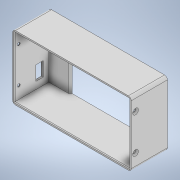
# Autodesk Inventor part: screen cover
Saved by Autodesk Inventor 2021 (Build 250183000, 183)
## iProperties
Created: 2022-01-29
Part Number: screen cover
Material: Generic
Document SubType Name: Modeling
Designer: Toby
Density: 1 g/cm^3
Appearance: Default
Author: Toby
Autodesk Inventor part; units mm, degrees
ref_plane "YZ Plane" through (0, 0, 0) normal (1, 0, 0) x (0, 1, 0)
ref_plane "XZ Plane" through (0, 0, 0) normal (0, 1, 0) x (-1, 0, 0)
ref_plane "XY Plane" through (0, 0, 0) normal (0, 0, 1) x (1, 0, 0)
sketch "Sketch1" plane through (0, 0, 0) normal (0, 0, 1) x (1, 0, 0)
  line L0 (-56.0804, 17.6748) -> (23.9196, 17.6748)
  line L1 (23.9196, 17.6748) -> (23.9196, -24.3252)
  line L2 (23.9196, -24.3252) -> (-56.0804, -24.3252)
  line L3 (-56.0804, -24.3252) -> (-56.0804, 17.6748)
  line L4 (-57.3304, 19.1748) -> (25.4196, 19.1748)
  line L5 (25.4196, 19.1748) -> (25.4196, -25.8252)
  line L6 (25.4196, -25.8252) -> (-57.3304, -25.8252)
  line L7 (-57.3304, -25.8252) -> (-57.3304, 19.1748)
  point P0 (0, 0)
  dimension "d0" = 80
  dimension "d1" = 42
  dimension "d2" = 1.5
  dimension "d3" = 1.5
  dimension "d4" = 1.25
  dimension "d5" = 1.5
  constraints: 16 end point, 4 parallel, 2 horizontal, 2 perpendicular
  measures "d0" distance of L0.start L0.end
  measures "d1" distance of L2.end L0.start
  measures "d2" distance between parallel lines of L0 L4
  measures "d3" distance between parallel lines of L6 L2
  measures "d4" distance between parallel lines of L7 L3
  measures "d5" distance between parallel lines of L1 L5
extrude "Extrusion1" add sketch "Sketch1" along normal blind 24
sketch "Sketch2" plane through (0, 0, 0) normal (0, 0, -1) x (-1, 0, 0)
  line L0 (-25.4196, -25.8252) -> (-25.4196, 19.1748) projected
  line L1 (57.3304, -25.8252) -> (-25.4196, -25.8252) projected
  line L2 (-25.4196, 19.1748) -> (57.3304, 19.1748)
  line L3 (57.3304, 19.1748) -> (57.3304, -25.8252)
  line L4 (57.3304, -25.8252) -> (-25.4196, -25.8252)
  line L5 (-25.4196, -25.8252) -> (-25.4196, 19.1748)
  point P0 (0, 0)
  constraints: 8 end point, 2 parallel, 1 horizontal, 1 perpendicular
extrude "Extrusion2" add sketch "Sketch2" along normal blind 1.2
fillet "Fillet1" radius 2 4 edges at (-57.3304, 19.1748, 11.4) (-57.3304, -25.8252, 11.4) (25.4196, -25.8252, 11.4) (25.4196, 19.1748, 11.4)
sketch "Sketch3" plane through (0, 0, 0) normal (0, 0, 1) x (1, 0, 0)
  line L0 (-56.0804, 17.6748) -> (23.9196, 17.6748) projected
  line L1 (-45.0804, 17.6748) -> (17.9196, 17.6748)
  line L2 (17.9196, 17.6748) -> (17.9196, -24.8955)
  line L3 (17.9196, -24.8955) -> (-45.0804, -24.8955)
  line L4 (-45.0804, -24.8955) -> (-45.0804, 17.6748)
  line L5 (23.9196, 17.6748) -> (23.9196, -24.3252) projected
  point P0 (0, 0)
  point P1 (17.9196, 17.6748)
  dimension "d11" = 6
  dimension "d12" = 69
  constraints: 8 end point, 2 parallel, 1 horizontal, 1 perpendicular, 1 point on line
  measures "d11" distance between parallel lines of L5 L2
  measures "d12" distance between parallel lines of L5 L4
extrude "Extrusion3" cut sketch "Sketch3" against normal blind 1.2
chamfer "Chamfer1" distance 1.2 angle 45 2 edges at (-45.0804, -3.3252, 0) (17.9196, -3.3252, 0)
sketch "Sketch4" plane through (-57.3304, -23.8252, 24) normal (-1, 0, 0) x (0, 0, 1)
  line L0 (-15, 14.5) -> (-20, 14.5)
  line L1 (-20, 14.5) -> (-20, 4.5)
  line L2 (-20, 4.5) -> (-15, 4.5)
  line L3 (-15, 4.5) -> (-15, 14.5)
  line L4 (-24, -0.5) -> (-24, 41.5) projected
  line L5 (-24, -0.5) -> (0, -0.5) projected
  point P0 (-24, 23.8252)
  dimension "d18" = 4
  dimension "d19" = 5
  dimension "d20" = 10
  dimension "d21" = 5
  constraints: 8 end point, 2 parallel, 1 horizontal, 1 perpendicular
  measures "d18" distance between parallel lines of L4 L1
  measures "d19" distance between parallel lines of L5 L2
  measures "d20" distance of L2.end L0.start
  measures "d21" distance between parallel lines of L1 L3
extrude "Extrusion4" cut sketch "Sketch4" against normal blind 1.5
sketch "Sketch5" plane through (-57.3304, -23.8252, 24) normal (-1, 0, 0) x (0, 0, 1)
  line L0 (0, 43) -> (-25.2, 43) projected
  line L1 (-25.2, -2) -> (0, -2) projected
  line L2 (0, 41) -> (0, 0) projected
  point P0 (-24, 23.8252)
  point P1 (-3, 33)
  point P2 (-3, 8)
  dimension "d24" = 10
  dimension "d25" = 10
  dimension "d26" = 3
  dimension "d27" = 3
  measures "d24" distance from line of L0 point (-3, 33)
  measures "d25" distance from line of L1 point (-3, 8)
  measures "d26" distance from line of L2 point (-3, 8)
  measures "d27" distance from line of L2 point (-3, 33)
hole "Hole1" at (-57.3304, 9.1748, 21) at (-57.3304, -15.8252, 21) direction (1, 0, 0) diameter 2 depth 10 tip angle 179 countersink diameter 4 countersink angle 90
sketch "Sketch6" plane through (25.4196, -23.8252, 24) normal (1, 0, 0) x (0, 0, -1)
  circle A0 centre (3, 8) radius 1 projected
  circle A1 centre (3, 33) radius 1 projected
  point P0 (24, 23.8252)
  constraints: 2 coincident
hole "Hole2" at (25.4196, -15.8252, 21) at (25.4196, 9.1748, 21) direction (-1, 0, 0) diameter 2 depth 10 tip angle 179 countersink diameter 4 countersink angle 90
sketch "Sketch7" plane through (0, 0, -1.2) normal (0, 0, -1) x (-1, 0, 0)
  line L0 (45.0804, -24.8955) -> (-17.9196, -24.8955) projected
  line L1 (-17.9196, -24.3252) -> (-17.9196, 17.6748) projected
  line L2 (45.0804, -24.8955) -> (-17.9196, -24.8955)
  line L3 (-17.9196, -24.8955) -> (-17.9196, -24.3252)
  line L4 (-17.9196, -24.3252) -> (45.0804, -24.3252)
  line L5 (45.0804, -24.3252) -> (45.0804, -24.8955)
  point P0 (0, 0)
  constraints: 8 end point, 2 parallel, 1 horizontal, 1 perpendicular
extrude "Extrusion5" add sketch "Sketch7" against normal blind 1.5
sketch "Sketch8" plane through (0, 0, -1.2) normal (0, 0, -1) x (-1, 0, 0)
  line L0 (-17.9196, -24.3252) -> (-17.9196, 17.6748) projected
  line L1 (-23.9196, -24.3252) -> (56.0804, -24.3252) projected
  line L2 (-17.9196, 17.6748) -> (41.0804, 17.6748)
  line L3 (41.0804, 17.6748) -> (41.0804, -24.3252)
  line L4 (41.0804, -24.3252) -> (-17.9196, -24.3252)
  line L5 (-17.9196, -24.3252) -> (-17.9196, 17.6748)
  line L6 (-23.9196, 17.6748) -> (-23.9196, -24.3252) projected
  line L7 (46.2804, -24.3252) -> (56.0804, -24.3252) projected
  line L8 (41.0804, 17.6748) -> (56.0804, 17.6748)
  line L9 (56.0804, 17.6748) -> (56.0804, -24.3252)
  line L10 (56.0804, -24.3252) -> (41.0804, -24.3252)
  line L11 (41.0804, -24.3252) -> (41.0804, 17.6748)
  point P0 (0, 0)
  dimension "d44" = 65
  constraints: 16 end point, 4 parallel, 2 horizontal, 2 perpendicular, 1 point on line
  measures "d44" distance between parallel lines of L6 L3
extrude "Extrusion6" add sketch "Sketch8" against normal blind 1.2 contours L3 L8 L9 L1
sketch "Sketch9" plane through (0, 0, -1.2) normal (0, 0, -1) x (-1, 0, 0)
  point P0 (0, 0)
chamfer "Chamfer2" distance 0.5 angle 45 4 edges at (-16.0804, 17.6748, 24) (-56.0804, -3.3252, 24) (-16.0804, -24.3252, 24) (23.9196, -3.3252, 24)
chamfer "Chamfer3" distance 1.2 angle 45 1 edges at (-41.0804, -3.3252, 0)
body "Solid1"
